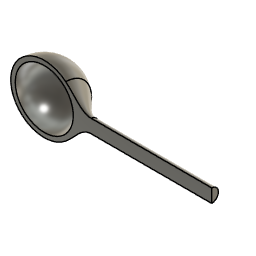
wind_speed_cup (Autodesk Fusion 360 design; units mm, degrees)
Autodesk Fusion 360 part; units mm, degrees
note: some values were not read from the file. Chosen so that the rebuilt part matches the saved one: a direction.
sketch "Szkic1" plane through (0, 0, 0) normal (0, 1, 0) x (1, 0, 0)
  line L0 (13, 0) -> (15, 0)
  line L1 (0, 0) -> (-15, 0)
  arc A0 (-15, 0) -> (15, 0) centre (0, 0) ccw
  arc A1 (-13, 0) -> (13, 0) centre (0, 0) ccw
  dimension "d1" = 30
  dimension "d2" = 26
  constraint coincident L1.start A0.centre
  constraint horizontal L0
  constraint parallel L0 L1
  constraint coincident L1 A1.start
  measures "d1" diameter of A0
  measures "d2" diameter of A1
revolve "Obrót1" add sketch "Szkic1" angle 180 about axis through (0, 0, 0) along (-1, 0, 0)
sketch "Szkic2" plane through (0, 0, 0) normal (0, 1, 0) x (1, 0, 0)
  line L0 (75, 0) -> (75, -3)
  line L1 (75, -3) -> (21, -3)
  spline S0 degree 5 poles (9.6157, -11.5125) (10.0753, -11.1286) (10.9799, -10.329) (12.293, -9.0341) (13.9792, -7.1799) (16.0934, -4.9797) (17.9027, -3.6587) (19.3902, -3.1198) (20.4518, -3) (21, -3) knots 0 0 0 0 0 0 0.2 0.4 0.6 0.8 1 1 1 1 1 1
  line L2 (8.6945, -12.2819) -> (10.5369, -10.7431)
  line L3 (20, -3) -> (22, -3)
  arc A0 (9.6157, -11.5125) -> (15, 0) centre (0, 0) ccw
  line L4 (15, 0) -> (75, 0)
  dimension "d9" = 60
  constraint vertical L0
  constraint horizontal L1
  constraint coincident A0.centre origin
  constraint midpoint S0.start L2
  constraint midpoint L1.end L3
  constraint coincident L1 L3.end
  constraint tangent L2 A0
  measures "d9" distance of A0.end L0.start
revolve "Obrót2" add sketch "Szkic2" angle 180 about axis through (1.75, 0, 0) along (-1, 0, 0) contours L0 L1 S0 L3 A0 L4
